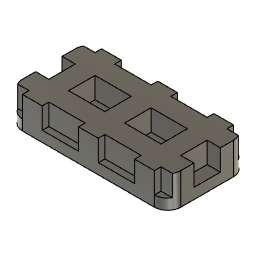
railCrossingPiece (Autodesk Fusion 360 archive; units mm, degrees)
design "railCrossing" references "TactileMapsParameters"
Autodesk Fusion 360 part; units mm, degrees
derive "ExternalDerived1" from "TactileMapsParameters v5"
sketch "Sketch1" plane through (0, 0, 0) normal (0, 0, 1) x (1, 0, 0)
  line L0 (0, 0) -> (12, 0)
  line L1 (12, 0) -> (12, 6)
  line L2 (12, 6) -> (0, 6)
  line L3 (0, 6) -> (0, 0)
  dimension "d18" = 12
  dimension "d19" = 6
  constraint horizontal L0
  constraint vertical L1
  constraint horizontal L2
  constraint vertical L3
  constraint coincident L0.start L3.end
  measures "d18" distance of L0.start L0.end
  measures "d19" distance of L0.start L2.end
extrude "Extrude1" add sketch "Sketch1" along normal blind 0.8
sketch "Sketch2" plane through (0, 0, 0.8) normal (0, 0, 1) x (-1, 0, 0)
  line L0 (0, -6) -> (0, 0)
  line L1 (0, 0) -> (-12, 0)
  line L2 (-12, 0) -> (-12, -6)
  line L3 (-12, -6) -> (0, -6)
  line L4 (0, -5.5) -> (-12, -5.5)
  line L5 (-12, -5.5) -> (-12, -4)
  line L6 (-12, -4) -> (0, -4)
  line L7 (0, -4) -> (0, -5.5)
  line L8 (0, -2) -> (-12, -2)
  line L9 (-12, -2) -> (-12, -0.5)
  line L10 (-12, -0.5) -> (0, -0.5)
  line L11 (0, -0.5) -> (0, -2)
  line L12 (-1, -6) -> (-2.5, -6)
  line L13 (-2.5, -6) -> (-2.5, 0)
  line L14 (-2.5, 0) -> (-1, 0)
  line L15 (-1, 0) -> (-1, -6)
  line L16 (-5.25, 0) -> (-5.25, -6)
  line L17 (-5.25, -6) -> (-6.75, -6)
  line L18 (-6.75, -6) -> (-6.75, 0)
  line L19 (-6.75, 0) -> (-5.25, 0)
  line L20 (-9.5, 0) -> (-9.5, -6)
  line L21 (-9.5, -6) -> (-11, -6)
  line L22 (-11, -6) -> (-11, 0)
  line L23 (-11, 0) -> (-9.5, 0)
  dimension "d22" = 12
  dimension "d23" = 1.5
  dimension "d24" = 0.5
  dimension "d25" = 12
  dimension "d26" = 1.5
  dimension "d27" = 2
  dimension "d28" = 1.5
  dimension "d29" = 6
  dimension "d30" = 1
  dimension "d33" = -4.25
  dimension "d34" = 0
  constraint horizontal L4
  constraint vertical L5
  constraint horizontal L6
  constraint vertical L7
  constraint coincident L0 L4.start
  constraint horizontal L8
  constraint vertical L9
  constraint horizontal L10
  constraint vertical L11
  constraint coincident L0 L8.start
  constraint horizontal L12
  constraint vertical L13
  constraint horizontal L14
  constraint vertical L15
  constraint coincident L3 L12.start
  measures "d22" distance of L4.start L4.end
  measures "d23" distance of L4.start L6.end
  measures "d24" distance of L3 L4
  measures "d25" distance of L8.start L8.end
  measures "d26" distance of L8.start L10.end
  measures "d27" distance of L6 L8
  measures "d28" distance of L12.start L12.end
  measures "d29" distance of L12.start L14.end
  measures "d30" distance of L7 L15
extrude "Extrude2" add sketch "Sketch2" along normal blind 1.6 contours L0 L4 L6 L7 L15 | L3 L4 L12 L13 L15 | L4 L6 L13 L15 | L0 L8 L10 L11 L15 | L6 L8 L13 L15 | L4 L6 L13 L16 | L3 L4 L16 L17 L18 | L8 L10 L13 L15 | L4 L6 L16 L18 | L1 L10 L13 L14 L15 | L8 L10 L13 L16 | L6 L8 L16 L18 | L4 L6 L18 L20 | L3 L4 L20 L21 L22 | L8 L10 L16 L18 | L4 L6 L20 L22 | L1 L10 L16 L18 L19 | L8 L10 L18 L20 | L6 L8 L20 L22 | L2 L4 L5 L6 L22 | L8 L10 L20 L22 | L1 L10 L20 L22 L23 | L2 L8 L9 L10 L22
fillet "Fillet1" radius 1 4 edges at (12, 0, 0.4) (0, 0, 0.4) (0, 6, 0.4) (12, 6, 0.4)
equation "length_Ref = 170 mm" comment "Side lengths of base of model"
equation "baseHeight_Ref = 0.4 mm" comment "Height of the base of the model"
equation "sidewalkHeight_Ref = 3.2 mm" comment "Height of sidewalk/walking surface"
equation "sidewalkWidth_Ref = length_Ref / 3" comment "Width of the sidewalk/walking surface"
equation "orientorSize_Ref = 6 mm" comment "Side length of orientation indicator square"
equation "oritentorHeight_Ref = 2.4 mm" comment "Height of the orientation indicator"
equation "braileHeight_Ref = 0.6 mm" comment "Standard height of Braille characters"
equation "filletRadius_Ref = 0.6 mm" comment "Radius of fillets to soften edges"
equation "lineWidth_Ref = 3 mm" comment "Width of crosswalk lines"
equation "lineHeight_Ref = braileHeight_Ref / 2" comment "Height of crosswalk lines"
equation "tabWidth_Ref = length_Ref / 10" comment "Width of tabs to secure adjacent maps together"
equation "tabLength_Ref = length_Ref / 14" comment "Length of tab to secure adjacent maps together"
equation "tabHeight_Ref = sidewalkHeight_Ref / 4" comment "Height of tabs to secure adjacent maps together"
equation "clearance_Ref = 0.4 mm" comment "Clearance around parts that will fit together"
equation "featureHeight_Ref = 1.6 mm" comment "Height of features such as bus stops"
equation "pegSize_Ref = 6 mm" comment "Side length of pegs/holes to connect features to map base"
equation "pegDepth_Ref = sidewalkHeight_Ref / 4" comment "Depth of pegs/holes to connect features to map base"
equation "d18 = 2 * pegSize_Ref"
equation "d19 = pegSize_Ref"
equation "d20 = pegDepth_Ref"
equation "d22 = pegSize_Ref * 2"
equation "d23 = pegSize_Ref / 4"
equation "d24 = pegSize_Ref / 12"
equation "d25 = 2 * pegSize_Ref"
equation "d26 = pegSize_Ref / 4"
equation "d27 = pegSize_Ref / 3"
equation "d28 = pegSize_Ref / 4"
equation "d29 = pegSize_Ref"
equation "d30 = pegSize_Ref / 6"
equation "d35 = featureHeight_Ref"
